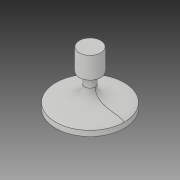
# Autodesk Inventor part: Top1
Saved by Autodesk Inventor 2018 (Build 220112000, 112)
## iProperties
Created: 2017-12-12
Part Number: Top1
Material: Generic
Document SubType Name: Modeling
Designer: Rus
Density: 1 g/cm^3
Appearance: Default
Author: Rus
Autodesk Inventor part; units mm, degrees
ref_plane "YZ Plane" through (0, 0, 0) normal (1, 0, 0) x (0, 1, 0)
ref_plane "XZ Plane" through (0, 0, 0) normal (0, 1, 0) x (-1, 0, 0)
ref_plane "XY Plane" through (0, 0, 0) normal (0, 0, 1) x (1, 0, 0)
sketch "Sketch1" plane through (0, 0, 0) normal (0, 0, 1) x (1, 0, 0)
  line L0 (0, 0) -> (0, 25.4)
  line L1 (0, 0) -> (0, -6.35)
  line L2 (0, 25.4) -> (0, 38.1)
  line L3 (6.35, 25.4) -> (6.35, 38.1)
  line L4 (6.35, 38.1) -> (0, 38.1)
  line L5 (3.175, 16.8251) -> (0, 16.8251) construction
  line L6 (6.35, 25.4) -> (3.175, 25.4)
  line L7 (3.175, 25.4) -> (0, 25.4) construction
  line L8 (0, 0) -> (3.175, 0) construction
  line L9 (3.175, 0) -> (18.1464, 0) construction
  line L10 (0, -6.35) -> (3.175, -4.2333)
  line L11 (3.175, -4.2333) -> (3.175, 0)
  line L12 (3.175, 25.4) -> (3.175, 19.05)
  arc A0 (6.0772, 2.8494) -> (3.175, 0) centre (6.0248, 0) ccw
  line L13 (3.175, 19.05) -> (3.175, 9.3106) construction
  line L14 (3.175, 9.3106) -> (16.4968, 12.5871) construction
  line L15 (16.4968, 12.5871) -> (20.32, 9.525) construction
  spline S0 degree 3 poles (3.175, 19.05) (3.175, 9.3106) (16.4968, 12.5871) (20.32, 9.525) knots 1 1 1 1 2 2 2 2
  line L16 (6.0772, 2.8494) -> (16.4968, 2.658) construction
  line L17 (16.4968, 2.658) -> (20.32, 6.35) construction
  spline S1 degree 2 poles (6.0772, 2.8494) (16.4968, 2.658) (20.32, 6.35) knots 1 1 1 2 2 2
  line L18 (20.32, 6.35) -> (20.32, 9.525)
  dimension "d5" = 44.45
  dimension "d6" = 12.7
  dimension "d7" = 6.35
  dimension "d12" = 2.1167
  dimension "d13" = 3.175
  dimension "d15" = 4.2333
  dimension "d31" = 6.35
  dimension "d33" = 20.32
  dimension "d34" = 6.35
  dimension "d35" = 3.175
  dimension "d36" = 3.175
  constraints: 30 end point, 8 vertical, 3 horizontal, 2 perpendicular, 2 point on circle, 2 point on line, 2 vertical alignment, 1 centre point, 1 tangent, 7 other
  measures "d5" distance of L2.end L1.end
  measures "d6" distance of L3.start L3.end
  measures "d7" distance between parallel lines of L2 L3
  measures "d12" vertical distance of L10.end L1.end
  measures "d13" horizontal distance of L1.end L10.end
  measures "d15" distance from line of L9 L10.end
  measures "d31" distance of L6.end L12.end
  measures "d33" distance between parallel lines of L0 L18
  measures "d34" distance from line of L8 L17.end
  measures "d35" distance of L17.end L15.end
  measures "d36" distance between parallel lines of L0 L12
revolve "Revolution1" add sketch "Sketch1" angle 360 about axis through (0, 25.4, 0) along (0, -1, 0)
body "Solid1"
